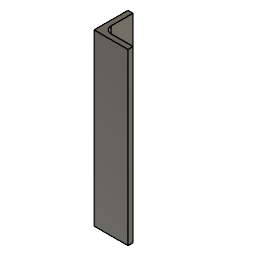
L-20×20×3 (Autodesk Fusion 360 design; units mm, degrees)
Autodesk Fusion 360 part; units mm, degrees
sketch "スケッチ1" plane through (0, 0, 0) normal (0, 0, 1) x (1, 0, 0)
  line L0 (0, 20) -> (0, 0)
  line L1 (3, 7) -> (3, 20)
  arc A0 (3, 7) -> (7, 3) centre (7, 7) ccw
  line L2 (0, 0) -> (20, 0)
  line L3 (20, 3) -> (7, 3)
  line L4 (20, 0) -> (20, 3)
  line L5 (3, 20) -> (0, 20)
extrude "押し出し1" add sketch "スケッチ1" along normal blind 100
